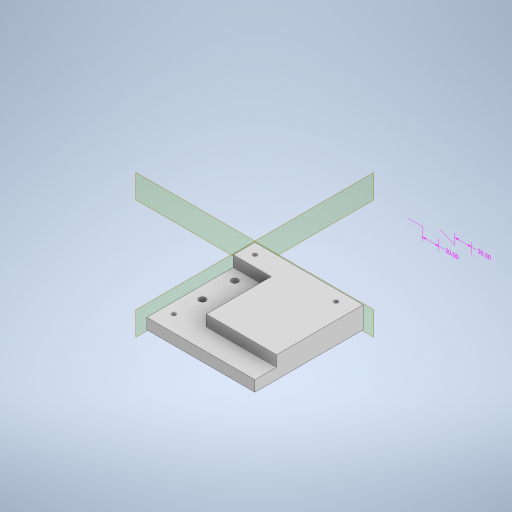
# Autodesk Inventor part: base_front_4
Saved by Autodesk Inventor 2023 (Build 270158000, 158)
## iProperties
Created: 2022-11-29
Part Number: base_front_4
Material: Genérico
Document SubType Name: Modeling
Designer: inigo
Density: 1 g/cm^3
Appearance: Valor por defecto
Author: inigo
Autodesk Inventor part; units mm, degrees
ref_plane "YZ Plane" through (0, 0, 0) normal (1, 0, 0) x (0, 1, 0)
ref_plane "XZ Plane" through (0, 0, 0) normal (0, 1, 0) x (-1, 0, 0)
ref_plane "XY Plane" through (0, 0, 0) normal (0, 0, 1) x (1, 0, 0)
sketch "Boceto1" plane through (0, 0, 0) normal (0, 1, 0) x (-1, 0, 0)
  line L0 (100, 100) -> (-100, 100)
  line L1 (-100, 100) -> (-100, -100)
  line L2 (-100, -100) -> (100, -100)
  line L3 (100, -100) -> (100, 100)
  line L4 (100, 100) -> (-100, -100) construction
  line L5 (-100, 100) -> (100, -100) construction
  point P0 (0, 0)
  dimension "d0" = 200
  dimension "d1" = 200
  constraints: 12 end point, 2 midpoint, 2 parallel, 1 horizontal, 1 perpendicular
  measures "d0" distance of L2.end L1.end
  measures "d1" distance of L1.end L0.end
extrude "Extrusión1" add sketch "Boceto1" along normal blind 20
sketch "Boceto2" plane through (0, 20, 0) normal (0, 1, 0) x (1, 0, 0)
  circle A0 centre (-11.5239, -30.0616) radius 3
  circle A1 centre (11.4761, -30.0616) radius 3
  circle A2 centre (-11.5239, -60.0616) radius 3
  circle A3 centre (11.4761, -60.0616) radius 3
  line L0 (-0.0239, -45.0616) -> (-35.0239, -45.0616)
  line L1 (-35.0239, -45.0616) -> (-35.0239, -80.0616)
  line L2 (-0.0239, -45.0616) -> (34.9761, -45.0616)
  line L3 (-11.5239, -30.0616) -> (11.4761, -60.0616)
  line L4 (-11.5239, -60.0616) -> (11.4761, -30.0616)
  line L5 (34.9761, -20.0616) -> (-35.0239, -20.0616)
  line L6 (-35.0239, -20.0616) -> (-35.0239, -80.0616)
  line L7 (34.9761, -80.0616) -> (34.9761, -20.0616)
  line L8 (-105, -100.0616) -> (105, -100.0616)
  line L9 (-105.0239, -80.0616) -> (104.9761, -80.0616)
  line L10 (-35.0239, -80.0616) -> (34.9761, -80.0616)
  line L11 (105, -100.0616) -> (95.8154, -100.0616)
  line L12 (-105.0239, -80.0616) -> (104.9761, -80.0616)
  line L13 (105, -80.0616) -> (-105, -80.0616)
  line L14 (-105, -100.0616) -> (105, -100.0616)
  line L15 (105, -90.0616) -> (94.0798, -90.0616)
  line L16 (-105, -100.0616) -> (105, -100.0616)
  line L17 (-105, -80.0616) -> (105, -80.0616)
  line L18 (105, -80.0616) -> (105, -100.0616)
  line L19 (105, -100.0616) -> (-105, -100.0616)
  line L20 (-105, -100.0616) -> (-105, -80.0616)
  line L21 (-100, 100) -> (-100, -100) projected
  line L22 (-100, -100) -> (100.4077, -100)
  point P0 (0, 0)
  point P1 (0, -10.0616)
  point P2 (0, -90.0616)
  point P3 (-0.0478, -80.0616)
  dimension "d4" = 20
  dimension "d5" = 20
  dimension "d6" = 30
  dimension "d7" = 30
  dimension "d8" = 20
  dimension "d9" = 35
  dimension "d10" = 35
  dimension "d11" = 60
  constraints: 40 end point, 5 equal length, 4 centre point, 3 perpendicular, 2 horizontal, 2 point on line, 1 midpoint, 6 other
  measures "d4" distance from line of L9 A2.centre
  measures "d5" distance from line of A3.centre L9
  measures "d6" distance between centres of A1 A3
  measures "d7" distance of A0.centre A2.centre
  measures "d8" distance between parallel lines of L8 L9
  measures "d9" distance of L2.start L2.end
  measures "d10" distance of L2.start L1.start
  measures "d11" distance of L7.end L7.start
extrude "Extrusión2" cut sketch "Boceto2" against normal blind 10
sketch "Boceto3" plane through (0, 20, 0) normal (0, 1, 0) x (1, 0, 0)
  circle A0 centre (-11.5239, -30.0616) radius 3 projected
  circle A1 centre (-11.5239, -30.0616) radius 3
  circle A2 centre (11.4761, -30.0616) radius 3 projected
  circle A3 centre (11.4761, -30.0616) radius 3
  circle A4 centre (11.4761, -60.0616) radius 3 projected
  circle A5 centre (11.4761, -60.0616) radius 3
  circle A6 centre (-11.5239, -60.0616) radius 3
  point P0 (0, 0)
  constraints: 4 centre point, 3 coincident
extrude "Extrusión3" cut sketch "Boceto3" against normal blind 20
sketch "Boceto4" plane through (0, 20, 0) normal (0, 1, 0) x (1, 0, 0)
  circle A0 centre (-51.75, 78.25) radius 1.75
  line L0 (-50, 70) -> (-60, 70)
  line L1 (-60, 70) -> (-60, 80)
  line L2 (-60, 80) -> (-50, 80)
  line L3 (-50, 80) -> (-50, 70)
  line L4 (-50, 70) -> (-60, 80) construction
  line L5 (-60, 70) -> (-50, 80) construction
  line L6 (-105, 90) -> (-105, -90)
  circle A1 centre (-58.25, 71.75) radius 1.75
  line L7 (0, 90) -> (0, 77.3124)
  circle A2 centre (51.75, 78.25) radius 1.75
  line L8 (50, 70) -> (60, 70)
  line L9 (60, 70) -> (60, 80)
  line L10 (60, 80) -> (50, 80)
  line L11 (50, 80) -> (50, 70)
  line L12 (50, 70) -> (60, 80) construction
  line L13 (60, 70) -> (50, 80) construction
  circle A3 centre (58.25, 71.75) radius 1.75
  line L14 (100, 100) -> (-100, 100) projected
  line L15 (-100, 100) -> (-100, -80.0616) projected
  line L16 (100, -80.0616) -> (100, 100) projected
  point P0 (0, 0)
  point P1 (0, 0)
  point P2 (-60, 75)
  point P3 (60, 75)
  dimension "d16" = 3.5
  dimension "d18" = 1.75
  dimension "d19" = 1.75
  dimension "d20" = 1.75
  dimension "d21" = 1.75
  dimension "d22" = 10
  dimension "d23" = 10
  dimension "d25" = 20
  dimension "d26" = 40
  dimension "d27" = 40
  constraints: 28 end point, 7 symmetric about line, 4 centre point, 2 parallel, 1 horizontal, 1 midpoint, 1 perpendicular, 1 vertical, 2 other
  measures "d16" diameter of A0
  measures "d18" distance from line of L2 A0.centre
  measures "d19" distance from line of L3 A0.centre
  measures "d20" distance from line of L1 A1.centre
  measures "d21" distance from line of L0 A1.centre
  measures "d22" distance between parallel lines of L0 L2
  measures "d23" distance between parallel lines of L3 L1
  measures "d25" distance between parallel lines of L14 L2
  measures "d26" distance between parallel lines of L1 L15
  measures "d27" distance between parallel lines of L16 L9
hole "Agujero1" at (-58.25, 20, -71.75) at (-51.75, 20, -78.25) at (58.25, 20, -71.75) at (51.75, 20, -78.25) direction (0, -1, 0) diameter 3.5 end through all
sketch "Boceto5" plane through (0, 20, 0) normal (0, 1, 0) x (1, 0, 0)
  line L0 (0, 90) -> (0, 68.25)
  circle A0 centre (-51.75, 78.25) radius 1.75 projected
  line L1 (-50, 78.25) -> (-50, 100)
  circle A1 centre (-58.25, 71.75) radius 1.75 projected
  line L2 (-60, 71.75) -> (-60, 100)
  line L3 (-60, 100) -> (-70, 100)
  line L4 (-50, 100) -> (-40, 100)
  line L5 (-40, 100) -> (-40, 60)
  line L6 (-40, 60) -> (-70, 60)
  line L7 (-70, 60) -> (-70, 100)
  line L8 (-70, 100) -> (-40, 100)
  circle A2 centre (51.75, 78.25) radius 1.75
  line L9 (50, 78.25) -> (50, 100)
  circle A3 centre (58.25, 71.75) radius 1.75
  line L10 (60, 71.75) -> (60, 100)
  line L11 (60, 100) -> (70, 100)
  line L12 (50, 100) -> (40, 100)
  line L13 (40, 100) -> (40, 60)
  line L14 (40, 60) -> (70, 60)
  line L15 (70, 60) -> (70, 100)
  line L16 (70, 100) -> (40, 100)
  point P0 (0, 0)
  dimension "d38" = 10
  dimension "d39" = 10
  dimension "d40" = 40
  constraints: 34 end point, 10 symmetric about line, 4 horizontal alignment, 4 vertical, 3 perpendicular, 6 other
  measures "d38" distance of L2.end L3.end
  measures "d39" distance of L1.end L4.end
  measures "d40" distance of L4.end L5.end
extrude "Extrusión4" cut sketch "Boceto5" against normal blind 10
ref_plane "Plano de trabajo1" through (0, 0, -100) normal (-1, 0, 0) x (0, 0, 1)
ref_plane "Plano de trabajo2" through (100, 0, 0) normal (0, 0, -1) x (-1, 0, 0)
sketch "Boceto7" plane through (0, 0, 0) normal (0, -1, 0) x (1, 0, 0)
  circle A0 centre (10, -10) radius 1.75
  line L0 (6.803, 0) -> (14.6069, 0)
  line L1 (0, 0) -> (0, -4.8284)
  line L2 (0, 0) -> (20.0354, 0)
  circle A1 centre (10, 10) radius 1.75
  line L3 (0, 0) -> (0, 4.8284)
  circle A2 centre (-10, -10) radius 1.75
  circle A3 centre (-10, 10) radius 1.75
  dimension "d52" = 3.5
  dimension "d54" = 10
  dimension "d55" = 10
  constraints: 8 end point, 4 centre point, 4 symmetric about line, 2 horizontal, 1 vertical, 3 other
  measures "d52" diameter of A0
  measures "d54" distance from line of L1 A0.centre
  measures "d55" distance from line of L2 A0.centre
hole "Agujero2" at (10, 0, -10) at (10, 0, 10) at (-10, 0, 10) at (-10, 0, -10) direction (0, 1, 0) diameter 3.5 end through all
sketch "Boceto8" plane through (0, 0, 0) normal (0, -1, 0) x (1, 0, 0)
  line L0 (-15, 15) -> (15, 15)
  line L1 (15, 15) -> (15, -15)
  line L2 (15, -15) -> (-15, -15)
  line L3 (-15, -15) -> (-15, 15)
  line L4 (-15, 15) -> (15, -15) construction
  line L5 (15, 15) -> (-15, -15) construction
  point P0 (0, 0)
  dimension "d63" = 30
  dimension "d64" = 30
  constraints: 12 end point, 2 midpoint, 2 parallel, 1 horizontal, 1 perpendicular
  measures "d63" distance of L1.end L2.end
  measures "d64" distance of L0.end L1.end
extrude "Extrusión5" cut sketch "Boceto8" against normal blind 10
sketch "Boceto9" plane through (0, 0, 0) normal (0, -1, 0) x (1, 0, 0)
  circle A0 centre (85, -10) radius 1.75
  line L0 (100, 100) -> (100, -100) projected
  line L1 (140, 0) -> (-140, 0) projected
  circle A1 centre (85, 10) radius 1.75
  line L2 (0, 0) -> (0, 9.4908)
  circle A2 centre (-85, -10) radius 1.75
  circle A3 centre (-85, 10) radius 1.75
  line L3 (0, 0) -> (6.3157, 6.3157)
  line L4 (0, 0) -> (8.9318, 0) construction
  circle A4 centre (10, 85) radius 1.75
  circle A5 centre (-10, -85) radius 1.75
  line L5 (0, 0) -> (5.9531, -5.9531)
  line L6 (0, 0) -> (8.419, 0) construction
  circle A6 centre (10, -85) radius 1.75
  circle A7 centre (-10, 85) radius 1.75
  dimension "d67" = 3.5
  dimension "d68" = 15
  dimension "d69" = 10
  dimension "d70" = 45
  dimension "d71" = 45
  constraints: 10 end point, 8 centre point, 7 symmetric about line, 2 equal length, 2 horizontal, 1 vertical, 7 other
  measures "d67" diameter of A0
  measures "d68" distance from line of L0 A0.centre
  measures "d69" distance from line of A0.centre L1
  measures "d70" angle of L4 L3
  measures "d71" angle of L5 L6
hole "Agujero3" at (-10, 0, 85) at (10, 0, 85) at (85, 0, 10) at (85, 0, -10) at (-85, 0, 10) at (-85, 0, -10) at (-10, 0, -85) at (10, 0, -85) direction (0, 1, 0) diameter 3.5 end through all
split "Dividir3" plane through (100, 0, 0) removes the side toward (0, 0, -1)
split "Dividir4" plane through (0, 0, -100) removes the side toward (-1, 0, 0)
